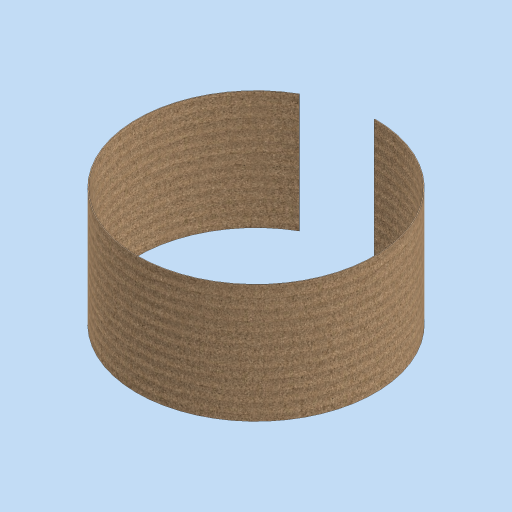
# Autodesk Inventor part: OBSTRUCCION_VISUAL
Saved by Autodesk Inventor 2024.2 (Build 282272000, 272)
## iProperties
Created: 2024-11-17
Part Number: OBSTRUCCION_VISUAL
Material: MDF Medium Density Fiberboard
Document SubType Name: Modeling
Designer: jrcer
Density: 0.8 g/cm^3
Appearance: Cardboard - Corrugated
Author: jrcer
Autodesk Inventor part; units mm, degrees
ref_plane "YZ Plane" through (0, 0, 0) normal (1, 0, 0) x (0, 1, 0)
ref_plane "XZ Plane" through (0, 0, 0) normal (0, 1, 0) x (-1, 0, 0)
ref_plane "XY Plane" through (0, 0, 0) normal (0, 0, 1) x (1, 0, 0)
sketch "Sketch1" plane through (0, 0, 0) normal (0, 1, 0) x (-1, 0, 0)
  circle A0 centre (0, 0) radius 70
  circle A1 centre (0, 0) radius 70.5
  line L0 (35, -60.6218) -> (35.25, -61.0548)
  line L1 (0, -70) -> (0, -70.5)
  line L2 (0, 0) -> (35.125, -60.8383) construction
  point P0 (0, -70.25)
  dimension "d0" = 140
  dimension "d1" = 141
  dimension "d4" = 30
  constraints: 6 end point, 4 point on circle, 2 centre point, 2 coincident, 2 midpoint, 1 collinear, 1 vertical, 1 vertical alignment
  measures "d0" diameter of A0
  measures "d1" diameter of A1
  measures "d4" angle of L2 L1
extrude "Extrusion1" add sketch "Sketch1" along normal blind 70 contours A0 L1 A1 L0 picked at (23.1516, 66.1792)
body "Solid1"
